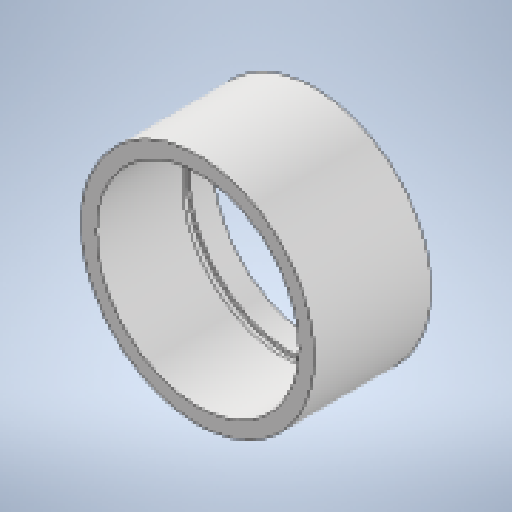
# Autodesk Inventor part: TRM 042 flange tube
Saved by Autodesk Inventor 2025.1 (Build 291241020, 241B)
## iProperties
Created: 2024-09-08
Part Number: TRM 042 flange tube
Material: Generic
Document SubType Name: Modeling
Designer: pokla
Density: 1 g/cm^3
Appearance: Default
Author: pokla
Autodesk Inventor part; units mm, degrees
ref_plane "YZ Plane" through (0, 0, 0) normal (1, 0, 0) x (0, 1, 0)
ref_plane "XZ Plane" through (0, 0, 0) normal (0, 1, 0) x (-1, 0, 0)
ref_plane "XY Plane" through (0, 0, 0) normal (0, 0, 1) x (1, 0, 0)
sketch "Sketch1" plane through (0, 0, 0) normal (0, 0, 1) x (1, 0, 0)
  line L0 (26, 0) -> (30, 0)
  line L1 (30, 0) -> (30, 30)
  line L2 (30, 30) -> (26, 30)
  line L3 (26, 30) -> (26, 0)
  line L4 (0, 0) -> (0, 24.4702) construction
  line L5 (26, 24) -> (27, 24)
  line L6 (27, 24) -> (27, 22)
  line L7 (27, 22) -> (26, 22)
  line L8 (26, 22) -> (26, 24)
  point P0 (28, 0)
  point P1 (26, 22)
  dimension "d0" = 4
  dimension "d1" = 30
  dimension "d2" = 52
  dimension "d4" = 2
  dimension "d5" = 6
  dimension "d6" = 1
  constraints: 18 end point, 4 parallel, 2 horizontal, 2 perpendicular, 1 horizontal alignment, 1 midpoint, 1 point on line, 1 vertical
  measures "d0" distance of L1.end L2.end
  measures "d1" distance of L0.end L1.end
  measures "d2" diameter of L0.start L4
  measures "d4" distance of L5.end L6.end
  measures "d5" distance of L5.start L2.end
  measures "d6" distance of L6.end L7.end
revolve "Revolution1" add sketch "Sketch1" angle 360 about axis through (0, 0, 0) along (0, 1, 0) contours L3 L7 L6 L5 L2 L1 L0
body "Solid1"
